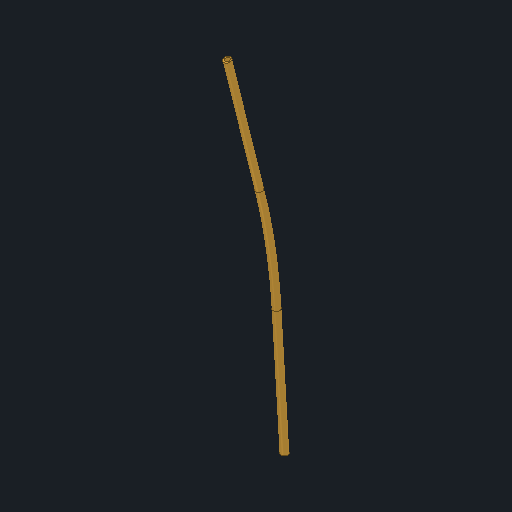
# Autodesk Inventor part: prop_shaft
Saved by Autodesk Inventor 2022.2 (Build 262287010, 287A)
## iProperties
Created: 2022-04-18
Part Number: prop_shaft
Material: Generic
Document SubType Name: Modeling
Designer: kardo
Density: 1 g/cm^3
Appearance: Brass - Prop shaft
Author: kardo
Autodesk Inventor part; units mm, degrees
ref_plane "YZ Plane" through (0, 0, 0) normal (1, 0, 0) x (0, 1, 0)
ref_plane "XZ Plane" through (0, 0, 0) normal (0, 1, 0) x (-1, 0, 0)
ref_plane "XY Plane" through (0, 0, 0) normal (0, 0, 1) x (1, 0, 0)
derived "stencil_frame.ipt"
sketch "sk_drivetrain_profile" plane through (6, 0, 0) normal (1, 0, 0) x (0, 1, 0)
  line L0 (-548.1262, 0) -> (397.7572, 0) construction
  line L1 (-363, 1541.8302) -> (-363, -1877.3857) construction
  line L2 (0, 1541.8302) -> (0, -1877.3857) construction
  line L3 (-140.12, 52.421) -> (-133.3462, 25.2528)
  line L4 (-388, 0) -> (-343.0839, 2.7472)
  line L5 (-136.7331, 38.8369) -> (-223.8252, 17.1224)
  line L6 (-300.1691, 5.372) -> (-261.4573, 7.7397) construction
  line L7 (-261.4573, 7.7397) -> (-223.8252, 17.1224) construction
  line L8 (-133.3462, 25.2528) -> (-133.3462, 20.2528) construction
  line L9 (-343.0839, 2.7472) -> (-300.1691, 5.372)
  line L10 (-513.6167, 1550.4344) -> (344.3546, -1890.7004) construction
  line L11 (-224.4013, 19.4329) -> (-137.3092, 41.1474) construction
  line L12 (-136.1571, 36.5264) -> (-223.2491, 14.8119) construction
  line L13 (-224.4013, 19.4329) -> (-223.2491, 14.8119) construction
  spline S0 degree 2 poles (-300.1691, 5.372) (-261.4573, 7.7397) (-223.8252, 17.1224) knots 1 1 1 2 2 2
  line L14 (0, 18.496) -> (-254.1001, 19.5569) construction
  line L15 (-55.187, 19.9264) -> (-309.3336, 20.9876) construction
  point P0 (0, 0)
  point P1 (-214.7203, 19.3925)
  point P2 (-205.0394, 19.3521)
  point P3 (-200.3057, 20.5323)
ref_plane "plane_motor_mount" through (0, -127.05, 0) normal (0, 0.9702957, 0.2419219) x (-1, 0, 0)
sketch "sk_prop_shaft_profile" plane through (0, -127.05, 0) normal (0, 0.9702957, 0.2419219) x (-1, 0, 0)
  circle A0 centre (-6, 40.0258) radius 2.3812
  point P0 (0, -30.7362)
  dimension "d1" = 4.7625
  constraints: 1 centre point, 1 coincident
  measures "d1" diameter of A0
derived "parameters_powertrain.ipt"
sweep "Sweep1" add profiles "sk_prop_shaft_profile" path "sk_drivetrain_profile" path curves L5 S0 L9 L4
shell "Shell1" thickness 0.7937 removed faces 2 at (6.4028, -388.0321, 0.5254) at (6.0476, -136.8279, 39.2169)
equation "\"d1\" = prop_shaft_od"
equation "\"prop_shaft_od\" = 4.7625"
body "Solid1"
